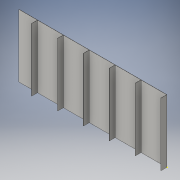
# Autodesk Inventor part: ModuleHolder
Saved by Autodesk Inventor 2016 (Build 200138000, 138)
## iProperties
Created: 2016-11-09
Part Number: ModuleHolder
Material: Generic
Document SubType Name: Modeling
Designer: RoboticsUser
Density: 1 g/cm^3
Appearance: Default
Mass: 5.51031 g
Surface Area: 435.598 cm^2
Volume: 5.51031 cm^3
Author: RoboticsUser
Autodesk Inventor part; units mm, degrees
ref_plane "YZ Plane" through (0, 0, 0) normal (1, 0, 0) x (0, 1, 0)
ref_plane "XZ Plane" through (0, 0, 0) normal (0, 1, 0) x (-1, 0, 0)
ref_plane "XY Plane" through (0, 0, 0) normal (0, 0, 1) x (1, 0, 0)
sketch "Sketch1" plane through (0, 0, 0) normal (0, 0, 1) x (1, 0, 0)
  line L0 (0, 0) -> (-203.2, 0)
  line L1 (-203.2, 0) -> (-203.2, 86.36)
  line L2 (-203.2, 86.36) -> (0, 86.36)
  line L3 (0, 86.36) -> (0, 0)
  dimension "d0" = 203.2
  dimension "d1" = 86.36
  constraints: 8 end point, 2 parallel, 1 horizontal, 1 perpendicular
  measures "d0" distance of L1.end L2.end
  measures "d1" distance of L0.end L1.end
extrude "Extrusion1" add sketch "Sketch1" along normal blind 0.254
sketch "Sketch2" plane through (0, 0, 0.254) normal (0, 0, 1) x (1, 0, 0)
  line L0 (-203.2, 0) -> (0, 0) projected
  line L1 (0, 0) -> (-0.254, 0)
  line L2 (-0.254, 0) -> (-0.254, 86.36)
  line L3 (-0.254, 86.36) -> (0, 86.36)
  line L4 (0, 86.36) -> (0, 0)
  dimension "d4" = 0.254
  constraints: 8 end point, 2 parallel, 1 horizontal, 1 perpendicular
  measures "d4" distance of L2.end L3.end
extrude "Extrusion2" add sketch "Sketch2" along normal blind 8.001
sketch "Sketch3" plane through (0, 0, 0) normal (1, 0, 0) x (0, 0, -1)
  point P0 (0, 0)
sketch "Sketch4" plane through (0, 0, 0.254) normal (0, 0, 1) x (1, 0, 0)
  line L0 (0, 0) -> (-203.2, 0) projected
  line L1 (-203.2, 86.36) -> (0, 86.36) projected
  line L2 (-35.56, 0) -> (-35.306, 0)
  line L3 (-35.306, 0) -> (-35.306, 86.36)
  line L4 (-35.306, 86.36) -> (-35.56, 86.36)
  line L5 (-35.56, 86.36) -> (-35.56, 0)
  dimension "d7" = 0.254
  constraints: 8 end point, 2 parallel, 2 point on line, 1 horizontal, 1 perpendicular
  measures "d7" distance of L4.end L3.end
extrude "Extrusion3" add sketch "Sketch4" along normal blind 8.001
sketch "Sketch5" plane through (0, 0, 0.254) normal (0, 0, 1) x (1, 0, 0)
  line L0 (0, 0) -> (-203.2, 0) projected
  line L1 (-203.2, 86.36) -> (0, 86.36) projected
  line L2 (-71.12, 0) -> (-70.866, 0)
  line L3 (-70.866, 0) -> (-70.866, 86.36)
  line L4 (-70.866, 86.36) -> (-71.12, 86.36)
  line L5 (-71.12, 86.36) -> (-71.12, 0)
  line L6 (-106.68, 0) -> (-106.426, 0)
  line L7 (-106.426, 0) -> (-106.426, 86.36)
  line L8 (-106.426, 86.36) -> (-106.68, 86.36)
  line L9 (-106.68, 86.36) -> (-106.68, 0)
  line L10 (-142.24, 0) -> (-141.986, 0)
  line L11 (-141.986, 0) -> (-141.986, 86.36)
  line L12 (-141.986, 86.36) -> (-142.24, 86.36)
  line L13 (-142.24, 86.36) -> (-142.24, 0)
  line L14 (-177.8, 0) -> (-177.546, 0)
  line L15 (-177.546, 0) -> (-177.546, 86.36)
  line L16 (-177.546, 86.36) -> (-177.8, 86.36)
  line L17 (-177.8, 86.36) -> (-177.8, 0)
  dimension "d10" = 0.254
  dimension "d11" = 0.254
  dimension "d12" = 0.254
  dimension "d13" = 0.254
  constraints: 32 end point, 8 parallel, 8 point on line, 4 horizontal, 4 perpendicular
  measures "d10" distance of L4.end L3.end
  measures "d11" distance of L8.end L7.end
  measures "d12" distance of L12.end L11.end
  measures "d13" distance of L16.end L15.end
extrude "Extrusion4" add sketch "Sketch5" along normal blind 8.001 contours L0 L5 L1 L3
sketch "Sketch6" plane through (0, 0, 0.254) normal (0, 0, 1) x (1, 0, 0)
  line L0 (0, 0) -> (-203.2, 0) projected
  line L1 (-203.2, 86.36) -> (0, 86.36) projected
  line L2 (-106.68, 0) -> (-106.426, 0)
  line L3 (-106.426, 0) -> (-106.426, 86.36)
  line L4 (-106.426, 86.36) -> (-106.68, 86.36)
  line L5 (-106.68, 86.36) -> (-106.68, 0)
  dimension "d16" = 0.254
  constraints: 8 end point, 2 parallel, 2 point on line, 1 horizontal, 1 perpendicular
  measures "d16" distance of L4.end L3.end
extrude "Extrusion5" add sketch "Sketch6" along normal blind 8.001
sketch "Sketch7" plane through (0, 0, 0.254) normal (0, 0, 1) x (1, 0, 0)
  line L0 (-203.2, 0) -> (-106.68, 0) projected
  line L1 (-106.68, 86.36) -> (-203.2, 86.36) projected
  line L2 (-142.24, 0) -> (-141.986, 0)
  line L3 (-141.986, 0) -> (-141.986, 86.36)
  line L4 (-141.986, 86.36) -> (-142.24, 86.36)
  line L5 (-142.24, 86.36) -> (-142.24, 0)
  point P0 (0, 0)
  dimension "d19" = 0.254
  constraints: 8 end point, 2 parallel, 2 point on line, 1 horizontal, 1 perpendicular
  measures "d19" distance of L4.end L3.end
extrude "Extrusion6" add sketch "Sketch7" along normal blind 8.001
sketch "Sketch8" plane through (0, 0, 0.254) normal (0, 0, 1) x (1, 0, 0)
  line L0 (0, 0) -> (-203.2, 0) projected
  line L1 (-203.2, 86.36) -> (0, 86.36) projected
  line L2 (-177.8, 0) -> (-177.546, 0)
  line L3 (-177.546, 0) -> (-177.546, 86.36)
  line L4 (-177.546, 86.36) -> (-177.8, 86.36)
  line L5 (-177.8, 86.36) -> (-177.8, 0)
  dimension "d22" = 0.254
  constraints: 8 end point, 2 parallel, 2 point on line, 1 horizontal, 1 perpendicular
  measures "d22" distance of L4.end L3.end
extrude "Extrusion7" add sketch "Sketch8" along normal blind 8.001
body "Solid1"
